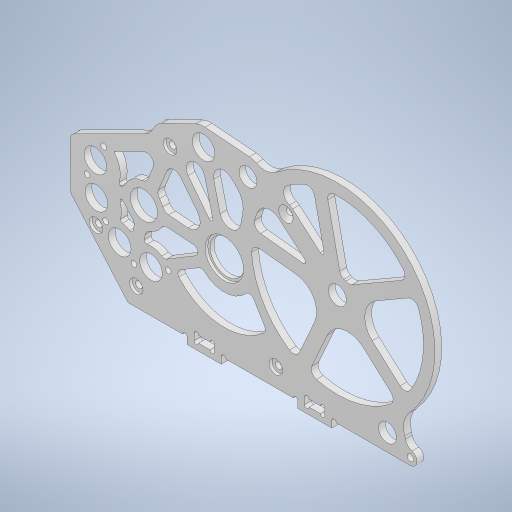
# Autodesk Inventor part: 主フレーム
Saved by Autodesk Inventor 2023 (Build 270158000, 158)
## iProperties
Created: 2022-06-18
Part Number: 主フレーム
Material: アルミニウム 2014-T6
Document SubType Name: Modeling
Designer: muzho
Density: 2.78927 g/cm^3
Appearance: サテン
Author: muzho
Autodesk Inventor part; units mm, degrees
ref_plane "YZ Plane" through (0, 0, 0) normal (1, 0, 0) x (0, 1, 0)
ref_plane "XZ Plane" through (0, 0, 0) normal (0, 1, 0) x (-1, 0, 0)
ref_plane "XY Plane" through (0, 0, 0) normal (0, 0, 1) x (1, 0, 0)
sketch "スケッチ5" plane through (0, 0, 0) normal (0, 0, 1) x (1, 0, 0)
  circle A0 centre (-51.0684, 48.1873) radius 1.3
  circle A1 centre (-58.3027, 33.9162) radius 1.3
  circle A2 centre (-50.1964, 20.1218) radius 1.3
  circle A3 centre (-37.7457, 10.0728) radius 1.3
  circle A4 centre (-22.565, 15.1272) radius 1.3
  circle A5 centre (-33.2954, 34.6933) radius 22.3153 construction
  circle A6 centre (2.1359, 32) radius 30.9835 construction
  circle A7 centre (52, 42.9528) radius 41.9528 construction
  circle A8 centre (2.1359, 32) radius 12.8528 construction
  circle A9 centre (-33.2954, 34.6933) radius 6.4335 construction
  circle A10 centre (-54.6856, 41.0518) radius 5.025
  circle A11 centre (-54.2496, 27.019) radius 5.025
  circle A12 centre (-43.9711, 15.0973) radius 5.025
  circle A13 centre (-30.1554, 12.6) radius 5.025
  circle A14 centre (-21.8214, 62.7533) radius 3
  circle A15 centre (-21.8214, 62.7533) radius 8
  line L0 (-21.8214, 62.7533) -> (-51.0684, 48.1873) construction
  line L1 (-33.3165, 55.1292) -> (-46.2281, 48.6988)
  arc A16 (-46.2281, 48.6988) -> (-46.7797, 47.8761) centre (-45.7823, 47.8037) ccw
  arc A17 (-52.9854, 52.0364) -> (-52.4722, 52.2518) centre (-51.0684, 48.1873) ccw construction
  arc A18 (-45.8061, 47.5867) -> (-65.5671, 39.279) centre (-54.6856, 41.0518) ccw construction
  line L2 (-65.7532, 43.7746) -> (-65.4452, 23.4769)
  arc A19 (-63.3575, 39.1831) -> (-63.6558, 28.9529) centre (-58.3027, 33.9162) ccw construction
  arc A20 (-45.2817, 33.4322) -> (-57.345, 16.4375) centre (-54.2496, 27.019) ccw construction
  arc A21 (-54.981, 15.674) -> (-41.5533, 4.3407) centre (-43.9711, 15.0973) ccw construction
  arc A22 (-65.4452, 23.4769) -> (-65.2027, 22.8391) centre (-64.4453, 23.4921) ccw
  line L3 (-65.2027, 22.8391) -> (-40.6377, -5.653)
  arc A23 (-40.6377, -5.653) -> (-39.8804, -6) centre (-39.8804, -5) ccw
  line L4 (-39.8804, -6) -> (84.0728, -6)
  line L5 (-6.7219, 36.0268) -> (-6.7219, -6.1434) construction
  line L6 (-37.0636, -3) -> (111.1776, -3) construction
  circle A24 centre (-10.2219, -3) radius 1
  circle A25 centre (-10.2219, -6) radius 1
  circle A26 centre (-15.2219, -6) radius 1
  line L7 (-11.2219, -3) -> (-11.2219, -6)
  circle A27 centre (-3.2219, -3) radius 1
  line L8 (-2.2219, -3) -> (-2.2219, -6)
  circle A28 centre (-3.2219, -6) radius 1
  circle A29 centre (1.7781, -6) radius 1
  line L9 (-9.2219, -3) -> (-4.2219, -3)
  line L10 (-14.2219, -6) -> (-14.2219, -9)
  line L11 (-14.2219, -9) -> (-7.7219, -9)
  line L12 (0.7781, -9) -> (-7.7219, -9)
  line L13 (0.7781, -6) -> (0.7781, -9)
  circle A30 centre (-33.2954, 34.6933) radius 6.025
  circle A31 centre (-33.2954, 34.6933) radius 9.025
  line L14 (-54.6856, 41.0518) -> (-54.2496, 27.019) construction
  line L15 (-54.4676, 34.0354) -> (-33.2954, 34.6933) construction
  arc A32 (-46.934, 49.3692) -> (-46.3247, 48.2383) centre (-44.0496, 50.1938) ccw
  arc A33 (-44.0483, 38.1537) -> (-46.3247, 48.2383) centre (-54.6856, 41.0518) ccw
  line L16 (-43.0524, 36.8913) -> (-44.0614, 36.8599)
  line L17 (-42.8971, 31.8937) -> (-43.9061, 31.8624)
  arc A34 (-44.0483, 38.1537) -> (-43.0524, 36.8913) centre (-43.0835, 37.8908) ccw
  arc A35 (-42.8971, 31.8937) -> (-43.8127, 30.5719) centre (-42.8661, 30.8942) ccw
  arc A36 (-43.5733, 24.2678) -> (-43.8127, 30.5719) centre (-54.2496, 27.019) ccw
  arc A37 (-43.5733, 24.2678) -> (-42.7563, 23.0298) centre (-42.605, 24.0183) ccw
  arc A38 (-39.5768, 21.8123) -> (-42.7563, 23.0298) centre (-43.9711, 15.0973) ccw
  arc A39 (-44.0614, 36.8599) -> (-41.4454, 38.5699) centre (-44.1545, 39.8585) ccw
  arc A40 (-41.189, 30.3181) -> (-43.9061, 31.8624) centre (-43.8129, 28.8638) ccw
  arc A41 (-39.5768, 21.8123) -> (-38.0451, 22.4712) centre (-39.0292, 22.649) ccw
  line L18 (-38.0451, 22.4712) -> (-37.6576, 24.615)
  line L19 (-43.9711, 15.0973) -> (-30.1554, 12.6) construction
  line L20 (-37.0632, 13.8486) -> (-33.2954, 34.6933) construction
  line L21 (-32.7374, 23.7256) -> (-33.1249, 21.5818)
  arc A42 (-33.1249, 21.5818) -> (-31.9208, 20.4284) centre (-32.1408, 21.4039) ccw
  arc A43 (-25.4967, 19.1343) -> (-31.9208, 20.4284) centre (-30.1554, 12.6) ccw
  arc A44 (-37.6576, 24.615) -> (-38.785, 27.5298) centre (-40.6098, 25.1486) ccw
  arc A45 (-30.6609, 26.0613) -> (-32.7374, 23.7256) centre (-29.7852, 23.192) ccw
  arc A46 (-32.898, 62.0405) -> (-29.1429, 65.9774) centre (-36.4645, 69.2016) ccw
  line L22 (-21.8214, 62.7533) -> (-33.2954, 34.6933) construction
  line L23 (-29.2023, 51.3083) -> (-31.562, 45.5374)
  line L24 (-23.2257, 52.7137) -> (-26.934, 43.645)
  arc A47 (-34.0785, 43.6842) -> (-31.562, 45.5374) centre (-34.3389, 46.6729) ccw
  arc A48 (-26.934, 43.645) -> (-26.437, 40.5595) centre (-24.1572, 42.5095) ccw
  arc A49 (-29.2023, 51.3083) -> (-33.3165, 55.1292) centre (-31.9791, 52.4438) ccw
  circle A50 centre (2.1359, 32) radius 7.5
  circle A51 centre (2.1359, 32) radius 8.5
  arc A52 (-25.4967, 19.1343) -> (-23.3056, 19.0484) centre (-24.3356, 20.7628) ccw
  line L25 (-23.3056, 19.0484) -> (-10.3971, 26.8036)
  line L26 (-30.1554, 12.6) -> (2.1359, 32) construction
  arc A53 (-24.9799, 38.2009) -> (-22.4432, 36.3756) centre (-22.2158, 39.3669) ccw
  arc A54 (-22.8222, 31.3899) -> (-25.6057, 29.969) centre (-23.0495, 28.3986) ccw
  line L27 (-22.4432, 36.3756) -> (-13.7997, 35.7185)
  line L28 (-22.8222, 31.3899) -> (-11.2755, 30.5122)
  line L29 (-33.2954, 34.6933) -> (2.1359, 32) construction
  arc A55 (-10.3971, 26.8036) -> (-11.2755, 30.5122) centre (-11.4271, 28.518) ccw
  circle A56 centre (-54.6856, 41.0518) radius 14 construction
  line L30 (42, 44.1233) -> (42, -23.5713) construction
  circle A57 centre (38.5, -3) radius 1
  circle A58 centre (38.5, -6) radius 1
  circle A59 centre (33.5, -6) radius 1
  line L31 (37.5, -3) -> (37.5, -6)
  line L32 (34.5, -6) -> (34.5, -9)
  line L33 (34.5, -9) -> (42, -9)
  circle A60 centre (45.5, -3) radius 1
  line L34 (46.5, -3) -> (46.5, -6)
  circle A61 centre (45.5, -6) radius 1
  line L35 (49.5, -6) -> (49.5, -9)
  line L36 (49.5, -9) -> (42, -9)
  circle A62 centre (50.5, -6) radius 1
  line L37 (39.5, -3) -> (44.5, -3)
  circle A63 centre (52, 42.9528) radius 4.025
  circle A64 centre (52, 42.9528) radius 8.025
  arc A65 (83.7206, 13.9916) -> (24.9838, 76.3454) centre (52, 42.9528) ccw
  line L38 (52, 42.9528) -> (49.2725, 42.9528) construction
  arc A66 (55.6469, 50.1013) -> (58.5102, 50.1755) centre (57.0102, 52.7736) ccw
  line L39 (58.5102, 50.1755) -> (80.3207, 62.7679)
  arc A67 (80.3207, 62.7679) -> (81.1227, 67.2896) centre (78.8207, 65.3659) ccw
  arc A68 (61.5102, 44.9794) -> (60.0142, 42.5368) centre (63.0102, 42.3813) ccw
  arc A69 (87.6377, 56.0054) -> (83.3207, 57.5717) centre (84.8207, 54.9736) ccw
  line L40 (61.5102, 44.9794) -> (83.3207, 57.5717)
  line L41 (52, 42.9528) -> (85.5729, 62.3361) construction
  line L42 (52, 42.9528) -> (90.7666, 42.9528) construction
  line L43 (47.1425, 51.3763) -> (41.9063, 76.0106)
  arc A70 (46.3283, 48.6302) -> (47.1425, 51.3763) centre (44.2081, 50.7526) ccw
  arc A71 (41.9063, 76.0106) -> (37.8537, 78.1706) centre (38.9719, 75.3868) ccw
  arc A72 (50.5989, 80.8797) -> (47.7752, 77.258) centre (50.7097, 77.8818) ccw
  line L44 (53.0114, 52.6238) -> (47.7752, 77.258)
  arc A73 (53.0114, 52.6238) -> (54.8721, 50.4462) centre (55.9458, 53.2475) ccw
  line L45 (42.4877, 40.936) -> (17.4411, 43.5686)
  arc A74 (44.8478, 39.3131) -> (42.4877, 40.936) centre (42.1741, 37.9525) ccw
  arc A75 (17.4411, 43.5686) -> (14.1344, 40.3818) centre (17.1275, 40.585) ccw
  arc A76 (15.4964, 53.3403) -> (18.0683, 49.5357) centre (18.3818, 52.5193) ccw
  line L46 (43.1149, 46.9032) -> (18.0683, 49.5357)
  arc A77 (43.1149, 46.9032) -> (45.7609, 48) centre (43.4285, 49.8867) ccw
  line L47 (50.9786, 33.2829) -> (40.7351, 10.2756)
  arc A78 (53.2514, 35.026) -> (50.9786, 33.2829) centre (53.7192, 32.0627) ccw
  arc A79 (40.7351, 10.2756) -> (42.7441, 6.146) centre (43.4757, 9.0554) ccw
  arc A80 (30.8406, 11.4457) -> (35.2538, 12.716) centre (32.5132, 13.9362) ccw
  line L48 (45.4973, 35.7233) -> (35.2538, 12.716)
  arc A81 (45.4973, 35.7233) -> (45.2719, 38.5787) centre (42.7567, 36.9435) ccw
  line L49 (60.881, 38.9932) -> (79.5968, 22.1414)
  arc A82 (59.9256, 41.6934) -> (60.881, 38.9932) centre (62.8884, 41.2226) ccw
  arc A83 (79.5968, 22.1414) -> (84.1451, 22.776) centre (81.6042, 24.3708) ccw
  arc A84 (75.4264, 13.0928) -> (75.582, 17.6825) centre (73.5746, 15.4531) ccw
  line L50 (56.8662, 34.5343) -> (75.582, 17.6825)
  arc A85 (56.8662, 34.5343) -> (54.0809, 35.2023) centre (54.8588, 32.3049) ccw
  circle A86 centre (52, 42.9528) radius 37.9528
  circle A87 centre (-36.6731, 2) radius 1.5
  circle A88 centre (-36.6731, 2) radius 3
  line L51 (-39.8804, -5) -> (-36.6731, 2) construction
  circle A89 centre (24.8719, 2) radius 1.5
  circle A90 centre (24.8719, 2) radius 3
  line L52 (24.8719, 10.9511) -> (24.8719, -6.9511) construction
  circle A91 centre (84.0728, -3) radius 1.5
  circle A92 centre (84.0728, -3) radius 3
  circle A93 centre (-7, 69.8979) radius 5.025
  circle A94 centre (-7, 69.8979) radius 8
  line L53 (-10.4739, 77.1043) -> (-25.2953, 69.9597)
  arc A95 (-10.262, 60.4449) -> (-3.6097, 60.4901) centre (-7, 69.8979) ccw construction
  line L54 (-6.4881, 59.2404) -> (-2.9595, 44.6027)
  line L55 (-7, 69.8979) -> (2.1359, 32) construction
  line L56 (-2.5409, 59.9345) -> (0.2846, 48.214)
  arc A96 (-17.1837, 53.5456) -> (-23.2257, 52.7137) centre (-19.9638, 51.3798) ccw
  line L57 (-21.8214, 62.7533) -> (2.1359, 32) construction
  line L58 (-17.1837, 53.5456) -> (-9.516, 43.7028)
  arc A97 (-13.7997, 35.7185) -> (-9.516, 43.7028) centre (-13.4242, 40.6583) ccw
  line L59 (-13.8028, 55.7144) -> (-4.5495, 43.8363)
  arc A98 (-4.5495, 43.8363) -> (-2.9595, 44.6027) centre (-3.8372, 44.3911) ccw
  arc A99 (0.2846, 48.214) -> (9.4313, 48.6842) centre (4.8139, 49.3059) ccw
  arc A100 (10.184, 52.7694) -> (9.4313, 48.6842) centre (52, 42.9528) ccw
  arc A101 (-6.6918, 22.6584) -> (11.7715, 23.4941) centre (2.1359, 32) ccw
  arc A102 (-6.6918, 22.6584) -> (-9.0955, 22.9192) centre (-8.0655, 21.2048) ccw
  line L60 (-9.0955, 22.9192) -> (-17.3907, 17.9356)
  arc A103 (-17.3907, 17.9356) -> (-17.8823, 14.9232) centre (-16.3608, 16.2212) ccw
  arc A104 (-20.5941, 11.3055) -> (-18.526, 16.6024) centre (-22.565, 15.1272) ccw construction
  arc A105 (-17.8823, 14.9232) -> (19.613, 12.3302) centre (2.1359, 32) ccw
  arc A106 (14.9853, 23.2005) -> (11.7715, 23.4941) centre (13.2709, 22.1705) ccw
  line L61 (14.9853, 23.2005) -> (19.9989, 14.8552)
  arc A107 (19.613, 12.3302) -> (19.9989, 14.8552) centre (18.2846, 13.8252) ccw
  arc A108 (10.184, 52.7694) -> (7.1716, 62.4577) centre (0.4487, 55.0548) ccw
  arc A109 (16.2511, 75.4723) -> (24.9838, 76.3454) centre (19.952, 82.5648) ccw
  line L62 (-6.3807, 77.8739) -> (13.1663, 76.3562)
  line L63 (5.0173, 64.4141) -> (7.1716, 62.4577)
  arc A110 (-6.4881, 59.2404) -> (-13.8028, 55.7144) centre (-10.5261, 58.267) ccw
  arc A111 (5.0173, 64.4141) -> (-2.5409, 59.9345) centre (1.9273, 61.0116) ccw
  circle A112 centre (29.2913, 62.5568) radius 1.5
  circle A113 centre (12.5499, 68.38) radius 4
  circle A114 centre (12.5499, 68.38) radius 8
  circle A115 centre (29.2913, 62.5568) radius 4.5
  line L64 (29.2913, 62.5568) -> (52, 42.9528) construction
  line L65 (26.3507, 59.1505) -> (37.7651, 49.2966)
  line L66 (32.2319, 65.9631) -> (44.4466, 55.4183)
  arc A116 (29.8767, 73.7907) -> (30.8356, 66.7835) centre (32.2084, 70.5405) ccw
  arc A117 (26.2931, 59.201) -> (16.7177, 56.9376) centre (22.2955, 54.7267) ccw
  arc A118 (37.0071, 47.5451) -> (37.7651, 49.2966) centre (37.1117, 48.5397) ccw
  arc A119 (44.4466, 55.4183) -> (46.0783, 56.3832) centre (45.1001, 56.1753) ccw
  circle A120 centre (74.0428, 1.5165) radius 4
  arc A121 (76.7818, -6) -> (71.3037, -6) centre (74.0428, 1.5165) ccw
  arc A122 (83.7206, 13.9916) -> (81.6262, 4.0643) centre (91.1055, 7.2491) ccw
  arc A123 (81.8996, 3.0231) -> (84.8251, -0.0958) centre (85.8281, 3.7764) ccw
  arc A124 (-64.0909, 46.5055) -> (-65.7532, 43.7746) centre (-62.7535, 43.8201) ccw
  line L67 (-64.0909, 46.5055) -> (-32.898, 62.0405)
  circle A125 centre (2.1359, 32) radius 11.5
  circle A126 centre (29.2913, 62.5568) radius 3.25
  circle A127 centre (-21.8214, 62.7533) radius 1.5
  circle A128 centre (-54.4309, 16.4709) radius 1.5
  circle A129 centre (-54.4309, 16.4709) radius 3
  arc A130 (-58.4163, 16.1295) -> (-54.5931, 12.4742) centre (-54.4309, 16.4709) ccw construction
  line L68 (-54.2496, 27.019) -> (-43.9711, 15.0973) construction
  line L69 (-54.4309, 16.4709) -> (-49.1103, 21.0581) construction
  arc A131 (68.9958, 49.3012) -> (67.3045, 33.2095) centre (73.9958, 40.6409) ccw
  arc A132 (63.2897, 28.7506) -> (47.4629, 25.3865) centre (56.5984, 21.3192) ccw
  arc A133 (41.9816, 27.827) -> (33.8915, 41.8396) centre (32.8462, 31.8943) ccw
  point P0 (0, 0)
  point P1 (0, 0)
  point P2 (-16.2219, -6)
  point P3 (0.7781, -6)
  point P4 (2.7781, -6)
  point P5 (32.5, -6)
  point P6 (51.5, -6)
  point P7 (-43.4211, 36.9495)
  point P8 (-46.5149, 48.4843)
  point P9 (-43.2615, 31.8127)
  point P10 (-4.2219, -6)
  point P11 (-9.2219, -6)
  point P12 (44.5, -6)
  point P13 (39.5, -6)
  point P14 (84.1451, 22.776)
  point P15 (14.1344, 40.3818)
  point P16 (44.8478, 39.3131)
  point P17 (45.2719, 38.5787)
  point P18 (30.8406, 11.4457)
  point P19 (42.7441, 6.146)
  point P20 (53.2514, 35.026)
  point P21 (54.0809, 35.2023)
  point P22 (75.4264, 13.0928)
  point P23 (50.5989, 80.8797)
  point P24 (81.3373, -1.7682)
  point P25 (33.8915, 41.8396)
  point P26 (41.9816, 27.827)
  point P27 (47.4629, 25.3865)
  point P28 (63.2897, 28.7506)
  dimension "d514" = 3
  dimension "d516" = 2
  dimension "d517" = 2
  dimension "d554" = 2
  dimension "d555" = 2
  dimension "d497" = 10.05
  dimension "d498" = 10.05
  dimension "d499" = 10.05
  dimension "d500" = 10.05
  dimension "d501" = 6
  dimension "d502" = 16
  dimension "d503" = 1
  dimension "d504" = 3
  dimension "d505" = 6
  dimension "d506" = 6
  dimension "d507" = 6
  dimension "d508" = 1
  dimension "d509" = 6
  dimension "d510" = 1
  dimension "d511" = 6
  dimension "d512" = 35.4313
  dimension "d513" = 8.8578
  dimension "d515" = 2
  dimension "d518" = 5
  dimension "d519" = 3.5
  dimension "d520" = 3
  dimension "d521" = 12.05
  dimension "d522" = 3
  dimension "d523" = 3
  dimension "d524" = 5
  dimension "d525" = 2.5
  dimension "d526" = 1
  dimension "d527" = 1
  dimension "d528" = 3
  dimension "d529" = 1
  dimension "d530" = 3
  dimension "d531" = 3
  dimension "d532" = 1
  dimension "d533" = 1
  dimension "d534" = 3
  dimension "d535" = 5
  dimension "d536" = 2.5
  dimension "d537" = 3
  dimension "d538" = 3
  dimension "d539" = 8
  dimension "d540" = 3
  dimension "d541" = 3
  dimension "d542" = 5
  dimension "d543" = 2.5
  dimension "d544" = 3
  dimension "d545" = 15
  dimension "d546" = 2
  dimension "d547" = 2
  dimension "d548" = 3
  dimension "d549" = 3
  dimension "d550" = 5
  dimension "d551" = 2.5
  dimension "d552" = 2
  dimension "d553" = 2
  dimension "d556" = 3.5
  dimension "d557" = 5
  dimension "d558" = 3
  dimension "d559" = 8.05
  dimension "d560" = 4
  dimension "d561" = 1
  dimension "d562" = 3
  dimension "d563" = 3
  dimension "d564" = 3
  dimension "d565" = 30
  constraints: 191 point on circle, 136 end point, 124 centre point, 103 tangent, 24 coincident, 20 parallel, 16 concentric, 14 symmetric about line, 11 vertical, 5 point on line, 4 horizontal, 4 midpoint, 3 perpendicular, 2 equal radius, 2 vertical alignment, 1 equal length, 199 other
  measures "d497" diameter of A10
  measures "d498" diameter of A11
  measures "d499" diameter of A12
  measures "d500" diameter of A13
  measures "d501" diameter of A14
  measures "d502" diameter of A15
  measures "d503" radius of A16
  measures "d504" radial gap between concentric circles of A0 A17
  measures "d505" radial gap between concentric circles of A10 A18
  measures "d506" radial gap between concentric circles of A1 A19
  measures "d507" radial gap between concentric circles of A20 A11
  measures "d508" radius of A22
  measures "d509" radial gap between concentric circles of A21 A12
  measures "d510" radius of A23
  measures "d512" horizontal distance of point (2.136, 32) A5.centre
  measures "d513" distance from line of point (2.136, 32) L5
  measures "d515" diameter of A24
  measures "d518" distance of point (-10.222, -6) point (-15.222, -6)
  measures "d519" distance from line of L5 A24.centre
  measures "d520" distance of L10.start L10.end
  measures "d521" diameter of A30
  measures "d523" radius of A32
  measures "d524" distance between parallel lines of L17 L16
  measures "d525" distance between parallel lines of L17 L15
  measures "d526" radius of A34
  measures "d527" radius of A35
  measures "d528" radial gap between concentric circles of A12 A38
  measures "d529" radius of A37
  measures "d530" radius of A39
  measures "d531" radius of A40
  measures "d532" radius of A41
  measures "d533" radius of A42
  measures "d534" radial gap between concentric circles of A13 A43
  measures "d535" distance between parallel lines of L21 L18
  measures "d536" distance between parallel lines of L20 L21
  measures "d537" radius of A45
  measures "d538" radius of A44
  measures "d539" radius of A46
  measures "d540" radius of A47
  measures "d541" radius of A48
  measures "d542" distance between parallel lines of L24 L23
  measures "d543" distance between parallel lines of L24 L22
  measures "d544" radius of A49
  measures "d545" diameter of A50
  measures "d546" radius of A52
  measures "d547" distance between parallel lines of L26 L25
  measures "d548" radius of A53
  measures "d549" radius of A54
  measures "d550" distance between parallel lines of L28 L27
  measures "d551" distance between parallel lines of L28 L29
  measures "d552" radius of A55
  measures "d553" diameter of A57
  measures "d556" distance from line of L30 A57.centre
  measures "d557" distance of point (38.5, -6) point (33.5, -6)
  measures "d558" distance of L32.start L32.end
  measures "d559" diameter of A63
  measures "d560" radial gap between concentric circles of A63 A64
  measures "d562" radius of A66
  measures "d563" radius of A67
  measures "d564" radius of A68
  measures "d565" angle of L42 L41
extrude "押し出し3" add sketch "スケッチ5" along normal blind 3 contours A15 | A15 L53 A94 A110 | A110 L59 A98 L54 A94 A111 L56 A99 A100 A108 A114 A109 A65 A122 A121 L4 A62 L34 A60 L37 A57 L31 A59 A29 L8 A27 L9 A24 L7 A26 A23 L3 A22 L2 A124 L67 A46 A15 | A94 | L62 A114 L63 A111 A94 | A114 | A31 | A121 L4 | A123 A92 A121 | A92 | A92 L4 A121 | L4 A25 A28 L13 L12 L11 L10 | L35 L36 L33 L32 L4 A58 A61 | A64 | A64 A66 L39 A67 A86 A69 L40 A68 | A68 L40 A131 L49 A82 A64 | A64 A70 L43 A71 A86 A72 L44 A73 | A82 L49 A83 A86 A84 L50 A85 A64 | A64 A77 L46 A118 L65 A115 L66 A119 L43 A70 | A85 L50 A132 L47 A78 A64 | A64 A74 L45 A75 A86 A76 L46 A77 | A78 L47 A79 A86 A80 L48 A81 A64 | A64 A81 L48 A133 L45 A74 | A115 | A116 A115 A117 A86 | A125 | A126
extrude "押し出し4" add sketch "スケッチ5" along normal blind 1.8 contours A14 | A51 | A88 | A90 | A129
chamfer "面取り1" distance 1.75 angle 45 1 edges at (27.7913, 62.5568, 3)
